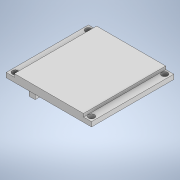
# Autodesk Inventor part: screen_footprint
Saved by Autodesk Inventor 2021 (Build 250183000, 183)
## iProperties
Created: 2021-12-12
Part Number: screen_footprint
Material: Generic
Document SubType Name: Modeling
Designer: Juan M. Casillas
Density: 1 g/cm^3
Appearance: Default
Author: Juan M. Casillas
Autodesk Inventor part; units mm, degrees
ref_plane "YZ Plane" through (0, 0, 0) normal (1, 0, 0) x (0, 1, 0)
ref_plane "XZ Plane" through (0, 0, 0) normal (0, 1, 0) x (-1, 0, 0)
ref_plane "XY Plane" through (0, 0, 0) normal (0, 0, 1) x (1, 0, 0)
sketch "Sketch1" plane through (0, 0, 0) normal (0, 1, 0) x (-1, 0, 0)
  line L0 (14, 13.5) -> (-14, 13.5)
  line L1 (-14, 13.5) -> (-14, -13.5)
  line L2 (-14, -13.5) -> (14, -13.5)
  line L3 (14, -13.5) -> (14, 13.5)
  line L4 (14, 13.5) -> (-14, -13.5) construction
  line L5 (-14, 13.5) -> (14, -13.5) construction
  line L6 (12.5, 12) -> (-12.5, 12)
  line L7 (-12.5, 12) -> (-12.5, -12)
  line L8 (-12.5, -12) -> (12.5, -12)
  line L9 (12.5, -12) -> (12.5, 12)
  point P0 (0, 0)
  dimension "d0" = 28
  dimension "d1" = 27
  dimension "d2" = 1.5
  constraints: 20 end point, 4 coincident, 4 parallel, 2 midpoint, 2 perpendicular, 1 horizontal, 3 other
  measures "d0" distance of L2.end L1.end
  measures "d1" distance of L1.end L0.end
  measures "d2" distance between parallel lines of L3 L9
extrude "Extrusion1" add sketch "Sketch1" against normal blind 1.5 contours L3 L2 L1 L0 | L9 L8 L7 L6
hole "Hole1" at (-12.5, 0, 12) at (-12.5, 0, -12) at (12.5, 0, -12) at (12.5, 0, 12) direction (0, -1, 0) diameter 2 end through all
sketch "Sketch2" plane through (0, 0, 0) normal (0, 1, 0) x (1, 0, 0)
  circle A0 centre (12.5, 12) radius 1 construction
  circle A1 centre (-12.5, -12) radius 1 construction
  circle A2 centre (-12.5, 12) radius 1 construction
  circle A3 centre (12.5, -12) radius 1 construction
  line L0 (14, -13.5) -> (14, 13.5) construction
  line L1 (14, 13.5) -> (-14, 13.5) construction
  line L2 (-14, 13.5) -> (-14, -13.5) construction
  line L3 (-14, -13.5) -> (14, -13.5) construction
  line L4 (-11.3162, -13.5) -> (11.3667, -13.5)
  line L5 (11.3667, -13.5) -> (11.3667, 13.5)
  line L6 (11.3667, 13.5) -> (-11.3162, 13.5)
  line L7 (-11.3162, 13.5) -> (-11.3162, -13.5)
  point P0 (0, 0)
  constraints: 8 end point, 2 parallel, 2 point on line, 1 horizontal, 1 perpendicular
extrude "Extrusion2" add sketch "Sketch2" along normal blind 1
sketch "Sketch3" plane through (0, -1.5, 0) normal (0, -1, 0) x (1, 0, 0)
  line L0 (-14, 6) -> (-12, 6)
  line L1 (-12, 6) -> (-12, -6)
  line L2 (-12, -6) -> (-14, -6)
  line L3 (-14, -6) -> (-14, 6)
  line L4 (-14, 6) -> (-12, -6) construction
  line L5 (-12, 6) -> (-14, -6) construction
  line L6 (-14, 13.5) -> (-14, -13.5) projected
  point P0 (0, 0)
  point P1 (-13, 0)
  point P2 (-14, 0)
  dimension "d14" = 2
  dimension "d15" = 12
  constraints: 12 end point, 4 midpoint, 2 parallel, 1 horizontal, 1 perpendicular
  measures "d14" distance of L2.end L1.end
  measures "d15" distance of L1.end L0.end
extrude "Extrusion3" add sketch "Sketch3" along normal blind 9
body "Solid1"
